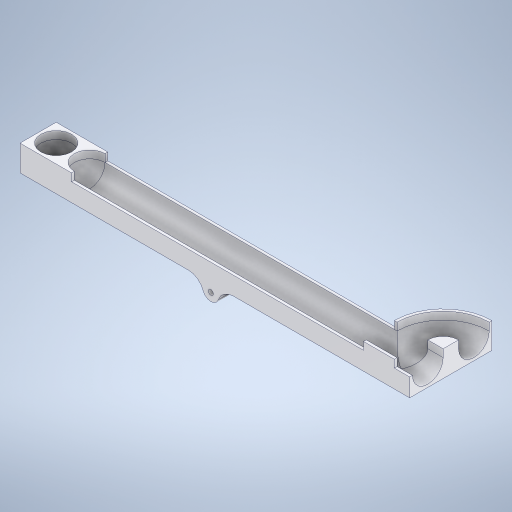
# Autodesk Inventor part: Trilho 5 min
Saved by Autodesk Inventor 2024 (Build 280153000, 153)
## iProperties
Created: 2023-05-15
Part Number: Trilho 5 min
Material: Plástico PET
Document SubType Name: Modeling
Designer: jpjoa
Density: 1.541 g/cm^3
Appearance: PTFE
Mass: 45.1122 g
Surface Area: 208.554 cm^2
Volume: 29.2746 cm^3
Author: jpjoa
Autodesk Inventor part; units mm, degrees
ref_plane "YZ Plane" through (0, 0, 0) normal (1, 0, 0) x (0, 1, 0)
ref_plane "XZ Plane" through (0, 0, 0) normal (0, 1, 0) x (-1, 0, 0)
ref_plane "XY Plane" through (0, 0, 0) normal (0, 0, 1) x (1, 0, 0)
sketch "Esboço1" plane through (0, 0, 0) normal (0, 1, 0) x (-1, 0, 0)
  arc A0 (-228.2, -28.6) -> (-219.2, -19.6) centre (-228.2, -19.6) ccw
  arc A1 (-228.2, -46.6) -> (-201.2, -19.6) centre (-228.2, -19.6) ccw
  line L0 (-201.2, -19.6) -> (-30.2, -19.6)
  line L1 (-219.2, -19.6) -> (-228.2, -19.6)
  line L2 (-228.2, -19.6) -> (-228.2, -1.6)
  line L3 (-228.2, -1.6) -> (-219.2, -1.6)
  line L4 (-219.2, -1.6) -> (-201.2, -1.6)
  line L5 (-201.2, -1.6) -> (-30.2, -1.6)
  arc A2 (-30.2, -19.6) -> (-30.2, -1.6) centre (-30.2, -10.6) ccw
  line L6 (-228.2, -28.6) -> (-228.2, -46.6)
  arc A3 (-228.2, -48.2) -> (-199.6448, -21.2) centre (-228.2, -19.6) ccw
  arc A4 (-228.2, -27) -> (-220.975, -21.2) centre (-228.2, -19.6) ccw
  line L7 (-220.975, -21.2) -> (-228.2, -21.2)
  line L8 (-228.2, 0) -> (-219.2, 0)
  line L9 (-219.2, 0) -> (-201.2, 0)
  line L10 (-201.2, 0) -> (0, 0)
  line L11 (0, -21.2) -> (-199.6448, -21.2)
  line L12 (-199.6448, -21.2) -> (-199.6448, -19.6)
  line L13 (-228.2, -46.6) -> (-228.2, -48.2)
  line L14 (-228.2, -28.6) -> (-228.2, -27)
  line L15 (-228.2, -21.2) -> (-228.2, -19.6)
  line L16 (-228.2, -1.6) -> (-228.2, 0)
  line L17 (-220.975, -21.2) -> (-220.975, -19.6)
  line L18 (-219.2, -1.6) -> (-219.2, 0)
  line L19 (-201.2, -1.6) -> (-201.2, 0)
  line L20 (0, -21.2) -> (0, 0)
  circle A5 centre (-10.6, -10.6) radius 9
  line L21 (-30.2, -21.2) -> (-30.2, -19.6)
  line L22 (-30.2, -1.6) -> (-30.2, 0)
  line L23 (-228.2, -21.2) -> (-228.2, -27)
  point P0 (-21.2, -10.6)
  point P1 (-30.2, -1.6)
  point P2 (-30.2, -19.6)
  dimension "d20" = 18
  dimension "d21" = 18
  dimension "d22" = 180
  dimension "d23" = 1.6
  dimension "d30" = 1.6
  dimension "d31" = 1.6
  dimension "d32" = 1.6
  dimension "d33" = 9
  dimension "d35" = 18
  dimension "d38" = 1.6
  dimension "d44" = 1.6
  dimension "d45" = 1.6
  constraints: 48 end point, 15 point on circle, 12 coincident, 12 point on line, 11 vertical, 11 vertical alignment, 7 horizontal alignment, 6 centre point, 2 horizontal, 2 tangent, 1 line through centre, 1 perpendicular, 1 other
  measures "d20" radial gap between concentric circles of A0 A1
  measures "d21" diameter of A2
  measures "d22" horizontal distance of point (-21.2, -10.6) L0.start
  measures "d23" radial gap between concentric circles of A1 A3
  measures "d30" distance between parallel lines of L11 L0
  measures "d31" radial gap between concentric circles of A0 A4
  measures "d32" distance between parallel lines of L1 L7
  measures "d33" distance of L1.start L1.end
  measures "d35" diameter of A5
  measures "d38" distance edge to line of A5 L20
  measures "d45" distance between parallel lines of L10 L5
extrude "Margem externa" add sketch "Esboço1" against normal blind 1.6 contours L14 A4 L17 L1 A0 | A0 L1 L2 L3 L4 L5 A2 L0 A1 L6 | A1 L0 L12 A3 L13 | L23 L7 A4 | L17 L7 L15 L1 | L0 L21 L11 L12 | L16 L8 L18 L3 | A2 L22 L10 L20 L11 L21 | L18 L9 L19 L4 | L5 L19 L10 L22 | A5
extrude "Proteção alta" add sketch "Esboço1" along normal blind 13.5 contours L14 A4 L17 L1 A0 | A1 L0 L12 A3 L13 | L23 L7 A4 | L17 L7 L15 L1 | A2 L22 L10 L20 L11 L21 | L18 L9 L19 L4
extrude "Proteção baixa" add sketch "Esboço1" along normal blind 9 contours L14 A4 L17 L1 A0 | A1 L0 L12 A3 L13 | L17 L7 L15 L1 | L0 L21 L11 L12 | L16 L8 L18 L3 | A2 L22 L10 L20 L11 L21 | L18 L9 L19 L4 | L5 L19 L10 L22
fillet "Arredondamento3" radius 9 7 edges at (19.6, 0, -10.6) (129.2, 0, -1.6) (115.7, 0, -19.6) (21.2, 0, -10.6) (209.1081, 0, -38.6919) (223.7, 0, -19.6) (221.836, 0, -25.964)
sketch "Esboço4" plane through (0, -1.6, 0) normal (0, -1, 0) x (1, 0, 0)
  line L0 (104.249, 0) -> (119.249, 0)
  line L1 (119.249, 0) -> (119.249, -10.6)
  line L2 (119.249, -10.6) -> (104.249, -10.6)
  line L3 (104.249, -10.6) -> (104.249, 0)
  line L4 (0, 0) -> (0, -21.2) projected
  point P0 (111.749, -10.6)
  point P1 (0, -10.6)
  point P2 (111.749, 0)
  dimension "d56" = 111.749
  dimension "d57" = 15
  constraints: 8 end point, 3 midpoint, 3 perpendicular, 2 horizontal alignment, 1 horizontal
  measures "d56" distance from line of L4 point (111.749, -10.6)
  measures "d57" distance of L0.start L0.end
extrude "Extrusão7" add sketch "Esboço4" along normal blind 9.4
sketch "Esboço5" plane through (119.249, -1.6, -10.6) normal (0, 0, -1) x (-1, 0, 0)
  circle A0 centre (7.5, -4.7) radius 1.5
  line L0 (0, 0) -> (0, -9.4) projected
  line L1 (15, -9.4) -> (0, -9.4) projected
  circle A1 centre (7.5, -4.7) radius 4.7
  line L2 (12.2, -4.7) -> (12.2, 0)
  line L3 (2.8, -4.7) -> (2.8, 0)
  line L4 (119.249, 0) -> (-80.3958, 0) projected
  line L5 (2.8, 0) -> (0, 0)
  line L6 (0, 0) -> (0, -9.4) projected
  line L7 (0, 0) -> (0, -9.4)
  line L8 (0, -9.4) -> (15, -9.4)
  line L9 (15, 0) -> (15, -9.4) projected
  line L10 (15, -9.4) -> (15, 0)
  line L11 (15, 0) -> (12.2, 0)
  point P0 (119.249, 1.6)
  point P1 (0, -4.7)
  point P2 (7.5, -9.4)
  point P3 (7.5, -9.4)
  dimension "d60" = 3
  dimension "d61" = 3.2
  constraints: 14 end point, 3 collinear, 3 vertical, 2 centre point, 2 midpoint, 2 point on circle, 2 point on line, 2 tangent, 1 horizontal alignment, 1 perpendicular, 1 vertical alignment
  measures "d60" diameter of A0
  measures "d61" radial gap between concentric circles of A0 A1
extrude "Extrusão8" cut sketch "Esboço5" against normal through all contours A0 | L4 L3 A1 L1 L0 | A1 L2 L4 L9 L1
fillet "Arredondamento5" radius 9 2 edges at (116.449, -1.6, -5.3) (107.049, -1.6, -5.3)
equation "\"d20\" = Esfera"
equation "\"d21\" = Esfera"
equation "\"d23\" = Margem"
equation "\"d30\" = Margem"
equation "\"d31\" = Margem"
equation "\"d28\" = Margem"
equation "\"d24\" = 0.75 * Esfera"
equation "\"Esfera\" = 18"
equation "\"Margem\" = 1.6"
equation "\"Furo\" = 3"
